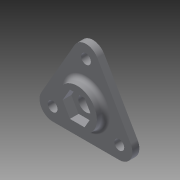
# Autodesk Inventor part: triangle_1
Saved by Autodesk Inventor 2013 (Build 170138000, 138)
## iProperties
Created: 2013-02-11
Part Number: triangle_1
Material: Generic
Document SubType Name: Modeling
Designer: Brad
Density: 1 g/cm^3
Author: Brad
Autodesk Inventor part; units mm, degrees
ref_plane "YZ Plane" through (0, 0, 0) normal (1, 0, 0) x (0, 1, 0)
ref_plane "XZ Plane" through (0, 0, 0) normal (0, 1, 0) x (-1, 0, 0)
ref_plane "XY Plane" through (0, 0, 0) normal (0, 0, 1) x (1, 0, 0)
sketch "Sketch1" plane through (0, 0, 0) normal (0, 0, 1) x (1, 0, 0)
  line L0 (0, 17.6092) -> (15.25, -8.8046)
  line L1 (15.25, -8.8046) -> (-15.25, -8.8046)
  line L2 (-15.25, -8.8046) -> (0, 17.6092)
  circle A0 centre (-15.25, -8.8046) radius 2.25
  circle A1 centre (15.25, -8.8046) radius 2.25
  circle A2 centre (0, 17.6092) radius 2.25
  circle A3 centre (0, 0) radius 3.5
  circle A4 centre (-15.25, -8.8046) radius 6
  circle A5 centre (15.25, -8.8046) radius 6
  circle A6 centre (0, 17.6092) radius 6
  line L3 (5.1962, 20.6092) -> (20.4462, -5.8046)
  line L4 (15.25, -14.8046) -> (-15.25, -14.8046)
  line L5 (-20.4462, -5.8046) -> (-5.1962, 20.6092)
  dimension "d7" = 30.5
  dimension "d8" = 4.5
  dimension "d11" = 360
  dimension "d13" = 7
  dimension "d14" = 12
  dimension "d17" = 360
  dimension "d19" = 6
  constraints: 12 end point, 7 centre point, 6 point on circle, 4 coincident, 21 other
  measures "d7" distance of L0.start L0.end
  measures "d8" diameter of A0
  measures "d13" diameter of A3
  measures "d14" diameter of A4
  measures "d19" distance between parallel lines of L2 L5
extrude "Extrusion1" add sketch "Sketch1" along normal blind 3.175 contours A2 L2 A6 L0 | L0 A6 L2 A2 | A6 L3 A5 L0 | L0 A5 L1 A4 L2 A6 | L2 A4 L5 A6 | A5 L1 A1 L0 | L0 A1 L1 A5 | A4 L1 A0 L2 | L2 A0 L1 A4 | A5 L4 A4 L1
sketch "Sketch2" plane through (0, 0, 0) normal (0, 0, -1) x (-1, 0, 0)
  circle A0 centre (0, 0) radius 3.5 projected
  circle A1 centre (0, 0) radius 6.5
  circle A2 centre (0, 0) radius 3.5
  dimension "d22" = 13
  constraints: 2 centre point, 2 coincident, 1 concentric
  measures "d22" diameter of A1
extrude "Extrusion2" add sketch "Sketch2" along normal blind 4.5
fillet "Fillet1" radius 3 1 edges at (6.5, 0, 0)
sketch "Sketch3" plane through (0, 0, 3.175) normal (0, 0, 1) x (1, 0, 0)
  circle A0 centre (0, 0) radius 3.5 projected
  line L0 (6.6973, 0) -> (3.3486, -5.8)
  line L1 (3.3486, -5.8) -> (-3.3486, -5.8)
  line L2 (-3.3486, -5.8) -> (-6.6973, 0)
  line L3 (-6.6973, 0) -> (-3.3486, 5.8)
  line L4 (-3.3486, 5.8) -> (3.3486, 5.8)
  line L5 (3.3486, 5.8) -> (6.6973, 0)
  circle A1 centre (0, 0) radius 9
  dimension "d26" = 11.6
  dimension "d27" = 18
  constraints: 12 end point, 2 coincident, 1 centre point, 13 other
  measures "d26" distance between parallel lines of L1 L4
  measures "d27" diameter of A1
extrude "Extrusion3" add sketch "Sketch3" along normal blind 4 contours A1
fillet "Fillet2" radius 2 1 edges at (-9, 0, 3.175)
body "Solid1"
